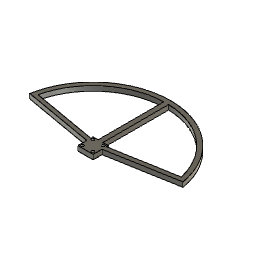
Prop_guard_hole v3 (Autodesk Fusion 360 design; units mm, degrees)
Autodesk Fusion 360 part; units mm, degrees
sketch "Sketch2" plane through (0, 0, 0) normal (0, 0, 1) x (1, 0, 0)
  line L0 (0, 0) -> (82, 0) construction
  line L1 (0, 0) -> (82, 0) construction
  arc A0 (80.7542, 14.2392) -> (-80.7542, 14.2392) centre (0, 0) ccw
  line L2 (-7.8232, -7.9921) -> (8.1768, -7.9921)
  circle A1 centre (-5.472, 5.4816) radius 1.5
  circle A2 centre (5.528, 5.4816) radius 1.5
  circle A3 centre (-5.472, -5.5184) radius 1.5
  circle A4 centre (5.528, -5.5184) radius 1.5
  line L3 (-75.3224, 17.4571) -> (-7.8232, 5.5552)
  line L4 (2.52, 77.3513) -> (2.52, 8.0079)
  line L5 (-2.5183, 8.0079) -> (-2.5183, 77.3462)
  line L6 (75.3853, 17.8691) -> (8.1768, 6.0184)
  arc A5 (75.3853, 17.8691) -> (2.52, 77.3513) centre (0.0798, -0.0088) ccw
  arc A6 (-2.5183, 77.3462) -> (-75.3224, 17.4571) centre (0.0798, -0.0088) ccw
  line L7 (76.2986, 13.4535) -> (80.7542, 14.2392)
  line L8 (8.1768, 1.4418) -> (76.2986, 13.4535)
  line L9 (-76.1439, 13.4262) -> (-80.7542, 14.2392)
  line L10 (-7.8232, 1.3794) -> (-76.1439, 13.4262)
  line L11 (-7.8232, 8.0079) -> (-7.8232, 5.5552)
  line L12 (-7.8232, 1.3794) -> (-7.8232, -7.9921)
  line L13 (8.1768, 8.0079) -> (2.52, 8.0079)
  line L14 (-2.5183, 8.0079) -> (-7.8232, 8.0079)
  line L15 (8.1768, -7.9921) -> (8.1768, 1.4418)
  line L16 (8.1768, 6.0184) -> (8.1768, 8.0079)
  dimension "d9" = 16
  dimension "d10" = 16
  dimension "d12" = 3
  dimension "d13" = 3
  dimension "d14" = 3
  dimension "d15" = 3
  constraint horizontal L0
  constraint horizontal L1
  constraint horizontal L2
  constraint vertical L15
  constraint horizontal L13
  constraint vertical L11
  constraint vertical L4
  constraint vertical L5
  constraint coincident L6.end L15
  constraint coincident L5.start L13
  constraint coincident L10.start L11
  measures "d9" distance of L2.start L2.end
  measures "d10" distance of L2.start L11.start
  measures "d12" diameter of A1
  measures "d13" diameter of A2
  measures "d14" diameter of A3
  measures "d15" diameter of A4
extrude "Extrude1" add sketch "Sketch2" along normal blind 5
